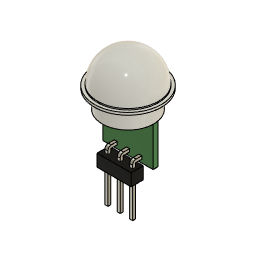
PIR Sensor (Autodesk Fusion 360 design; units mm, degrees)
Autodesk Fusion 360 part; units mm, degrees
note: some values were not read from the file. Chosen so that the rebuilt part matches the saved one: which bodies a step acts on; where a step starts.
sketch "Sketch1" plane through (0, 0, 0) normal (0, 1, 0) x (1, 0, 0)
  line L0 (5.15, 4.1) -> (-5.15, 4.1)
  line L1 (-5.15, 4.1) -> (-5.15, -4.1)
  line L2 (-5.15, -4.1) -> (5.15, -4.1)
  line L3 (5.15, -4.1) -> (5.15, 4.1)
  line L4 (5.15, 4.1) -> (-5.15, -4.1) construction
  line L5 (-5.15, 4.1) -> (5.15, -4.1) construction
  line L6 (-2.2385, 3.3985) -> (-2.8415, 3.3985)
  line L7 (-2.8415, 3.3985) -> (-2.8415, 2.8015)
  line L8 (-2.8415, 2.8015) -> (-2.2385, 2.8015)
  line L9 (-2.2385, 2.8015) -> (-2.2385, 3.3985)
  line L10 (-2.2385, 3.3985) -> (-2.8415, 2.8015) construction
  line L11 (-2.8415, 3.3985) -> (-2.2385, 2.8015) construction
  line L12 (0.3, 3.4) -> (-0.3, 3.4)
  line L13 (-0.3, 3.4) -> (-0.3, 2.8)
  line L14 (-0.3, 2.8) -> (0.3, 2.8)
  line L15 (0.3, 2.8) -> (0.3, 3.4)
  line L16 (0.3, 3.4) -> (-0.3, 2.8) construction
  line L17 (-0.3, 3.4) -> (0.3, 2.8) construction
  line L18 (2.84, 3.4) -> (2.24, 3.4)
  line L19 (2.24, 3.4) -> (2.24, 2.8)
  line L20 (2.24, 2.8) -> (2.84, 2.8)
  line L21 (2.84, 2.8) -> (2.84, 3.4)
  line L22 (2.84, 3.4) -> (2.24, 2.8) construction
  line L23 (2.24, 3.4) -> (2.84, 2.8) construction
  point P0 (-2.54, 3.1)
  point P1 (0, 3.1)
  point P2 (2.54, 3.1)
  dimension "d1" = 10.3
  dimension "d2" = 8.2
  dimension "d5" = 2.54
  dimension "d7" = 2.54
  dimension "d8" = 1
  constraint perpendicular L0 L1
  constraint parallel L0 L2
  constraint parallel L1 L3
  constraint horizontal L0
  constraint coincident L4 origin
  constraint coincident L5 origin
  constraint perpendicular L6 L7
  constraint parallel L6 L8
  constraint parallel L7 L9
  constraint horizontal L6
  constraint coincident L10 P0
  constraint coincident L11 P0
  constraint perpendicular L12 L13
  constraint parallel L12 L14
  constraint parallel L13 L15
  constraint horizontal L12
  constraint coincident L16 P1
  constraint coincident L17 P1
  constraint perpendicular L18 L19
  constraint parallel L18 L20
  constraint parallel L19 L21
  constraint horizontal L18
  constraint coincident L22 P2
  constraint coincident L23 P2
  measures "d1" distance of L1.end L2.end
  measures "d2" distance of L0.end L1.end
  measures "d5" distance of P1 P2
  measures "d7" distance of P0 P1
  measures "d8" distance of L0 P0
sketch "Sketch2" plane through (0, 0, 0) normal (1, 0, 0) x (0, 1, 0)
  line L0 (0, -3.1) -> (2, -3.1)
  line L1 (0, -3.1) -> (-1.19, -3.1)
  line L2 (-1.6, -3.51) -> (-1.6, -13.4)
  arc A0 (-1.19, -3.1) -> (-1.6, -3.51) centre (-1.19, -3.51) ccw
  point P0 (-1.6, -3.1)
  dimension "d9" = 2
  dimension "d10" = 1.6
  dimension "d11" = 10.3
  dimension "d12" = 0.41
  constraint horizontal L0
  constraint parallel L0 L1
  constraint perpendicular L1 L2
  constraint coincident P0 L2
  constraint coincident P0 L1
  constraint tangent L2 A0
  constraint tangent L1 A0
  measures "d9" distance of L0.start L0.end
  measures "d10" distance of L0.start P0
  measures "d11" distance of P0 L2.end
  measures "d12" radius of A0
sweep "Sweep1" add profiles "Sketch1" path "Sketch2" along L0 L1 A0 L2 section 1 contours L6 L7 L8 L9 | L12 L13 L14 L15 | L18 L19 L20 L21 makes body 1 at (-0.3, -1.5, -6.8067) makes body 2 at (2.24, -1.5, -6.8067) makes body 3 at (-2.8415, -1.5005, -6.8067)
sketch "Sketch3" plane through (0, 0, 0) normal (1, 0, 0) x (0, 1, 0)
  line L0 (-2.8583, -6.5672) -> (-0.3583, -6.5672)
  line L1 (-0.3583, -6.5672) -> (-0.3583, -4.0672)
  line L2 (-0.3583, -4.0672) -> (-2.8583, -4.0672)
  line L3 (-2.8583, -4.0672) -> (-2.8583, -6.5672)
  line L4 (-2.8583, -6.5672) -> (-0.3583, -4.0672) construction
  line L5 (-0.3583, -6.5672) -> (-2.8583, -4.0672) construction
  point P0 (-1.6083, -5.3172)
  dimension "d19" = 2.5
  dimension "d20" = 2.5
  constraint perpendicular L0 L1
  constraint parallel L0 L2
  constraint parallel L1 L3
  constraint horizontal L0
  constraint coincident L4 P0
  constraint coincident L5 P0
  measures "d19" distance of L0.end L1.end
  measures "d20" distance of L1.end L2.end
extrude "Extrude1" add sketch "Sketch3" along normal mid plane 7 separate body makes body 4
extrude "Extrude2" add sketch "Sketch1" along normal blind 1 separate body makes body 5
sketch "Sketch4" plane through (0, 0, 0) normal (0, 0, 1) x (1, 0, 0)
  circle A0 centre (0, 0) radius 5.3
  circle A1 centre (0, 0) radius 6.25
  circle A2 centre (0, 0) radius 4.7
  circle A3 centre (0, 0) radius 6.875
  dimension "d25" = 10.6
  dimension "d27" = 12.5
  dimension "d28" = 0.6
  dimension "d44" = 13.75
  constraint coincident A0.centre A1.centre
  constraint concentric A1 A3
  measures "d25" diameter of A0
  measures "d27" diameter of A1
  measures "d44" diameter of A3
extrude "Extrude3" add sketch "Sketch4" along normal blind 4.5 from surface at 4.1 separate body contours A2 makes body 6
extrude "Extrude4" add sketch "Sketch4" along normal blind 6 from surface at 4.1 separate body contours A0 makes body 7
extrude "Extrude5" add sketch "Sketch4" along normal blind 0.5 from surface at 7.85 contours A1 | A3 bodies 7
extrude "Extrude6" add sketch "Sketch4" along normal blind 6.5 from surface at 8.35 separate body contours A0 | A1 | A2 makes body 9
fillet "Fillet1" radius 6.25 1 edges at (-5.827, -2.2601, 14.85) on bodies 9
shell "Shell1" thickness 0.49 removed faces 1 at (0.0274, -1.4841, 8.35) on bodies 9
copy_body "Body->Comp1" bodies 3 removing the originals makes body 10 in component "Legs"
copy_body "CutPasteBodies1" bodies 1 2 4 removing the originals makes body 11 makes body 12 makes body 13 in component "Legs"
copy_body "CutPasteBodies1'" bodies 9 removing the originals makes body 14 in component "Cap"
copy_body "CutPasteBodies2" bodies 7 removing the originals makes body 15 in component "Cap"
copy_body "CutPasteBodies3" bodies 6 removing the originals makes body 16 in component "Cap"
copy_body "CutPasteBodies1''" bodies 5 removing the originals makes body 17 in component "Board"
component "Legs" placed x (1, 0, 0) y (0, 1, 0) z (0, 0, 1) at (0, 0, 0)
component "Board" placed x (1, 0, 0) y (0, 1, 0) z (0, 0, 1) at (0, 0, 0)
component "Cap" placed x (1, 0, 0) y (0, 1, 0) z (0, 0, 1) at (0, 0, 0)
